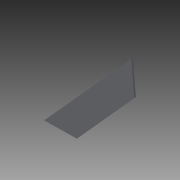
# Autodesk Inventor part: End Polycarbonate 125
Saved by Autodesk Inventor 2015 (Build 190159000, 159)
## iProperties
Created: 2015-01-21
Part Number: End Polycarbonate 125
Material: Generic
Document SubType Name: Modeling
Designer: peters
Density: 1 g/cm^3
Appearance: Default
Author: peters
Autodesk Inventor part; units mm, degrees
ref_plane "YZ Plane" through (0, 0, 0) normal (1, 0, 0) x (0, 1, 0)
ref_plane "XZ Plane" through (0, 0, 0) normal (0, 1, 0) x (-1, 0, 0)
ref_plane "XY Plane" through (0, 0, 0) normal (0, 0, 1) x (1, 0, 0)
sketch "Sketch1" plane through (0, 0, 0) normal (0, 0, 1) x (1, 0, 0)
  line L0 (193.5851, 2.9523) -> (0, 0)
  line L1 (533.5951, 380.3872) -> (193.5851, 2.9523)
  line L2 (533.5951, 380.3872) -> (516.3897, 573.2288)
  line L3 (0, 0) -> (193.5851, 2.9523)
  line L4 (193.5851, 2.9523) -> (533.5951, 380.3872)
  line L5 (533.5951, 380.3872) -> (516.3897, 573.2288)
  line L6 (516.3897, 573.2288) -> (0, 0)
  point P0 (0, 0)
  constraints: 14 end point, 2 collinear, 1 parallel
extrude "Extrusion1" add sketch "Sketch1" along normal blind 9.525
body "Solid1"
